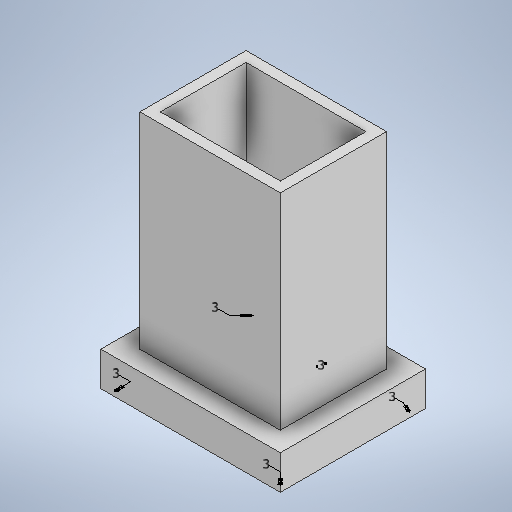
# Autodesk Inventor part: Part3
Saved by Autodesk Inventor 2025.3 (Build 293356000, 356)
## iProperties
Created: 2026-04-30
Part Number: Part3
Material: Generic
Document SubType Name: Modeling
Designer: kamal
Density: 1 g/cm^3
Appearance: Default
Author: kamal
Autodesk Inventor part; units mm, degrees
ref_plane "YZ Plane" through (0, 0, 0) normal (1, 0, 0) x (0, 1, 0)
ref_plane "XZ Plane" through (0, 0, 0) normal (0, 1, 0) x (-1, 0, 0)
ref_plane "XY Plane" through (0, 0, 0) normal (0, 0, 1) x (1, 0, 0)
sketch "Sketch1" plane through (0, 0, 0) normal (0, 1, 0) x (-1, 0, 0)
  line L0 (-17.5, 12.5) -> (17.5, 12.5)
  line L1 (17.5, 12.5) -> (17.5, -12.5)
  line L2 (17.5, -12.5) -> (-17.5, -12.5)
  line L3 (-17.5, -12.5) -> (-17.5, 12.5)
  line L4 (-17.5, 12.5) -> (17.5, -12.5) construction
  line L5 (17.5, 12.5) -> (-17.5, -12.5) construction
  line L6 (26.2, -21.2) -> (-26.2, -21.2)
  line L7 (-26.2, -21.2) -> (-26.2, 21.2)
  line L8 (-26.2, 21.2) -> (26.2, 21.2)
  line L9 (26.2, 21.2) -> (26.2, -21.2)
  line L10 (26.2, -21.2) -> (-26.2, 21.2) construction
  line L11 (-26.2, -21.2) -> (26.2, 21.2) construction
  line L12 (20.5, 15.5) -> (-20.5, 15.5)
  line L13 (-20.5, 15.5) -> (-20.5, -15.5)
  line L14 (-20.5, -15.5) -> (20.5, -15.5)
  line L15 (20.5, -15.5) -> (20.5, 15.5)
  point P0 (0, 0)
  dimension "d0" = 35
  dimension "d1" = 25
  dimension "d2" = 52.4
  dimension "d3" = 42.4
  dimension "d4" = 3
  constraints: 32 end point, 6 parallel, 4 midpoint, 3 perpendicular, 2 horizontal, 3 other
  measures "d0" distance of L1.end L2.end
  measures "d1" distance of L0.end L1.end
  measures "d2" distance of L7.end L8.end
  measures "d3" distance of L8.end L6.start
  measures "d4" distance between parallel lines of L0 L12
extrude "Extrusion1" add sketch "Sketch1" along normal blind 60 contours L15 L14 L13 L12
extrude "Extrusion2" add sketch "Sketch1" against normal blind 10 contours L6 L7 L8 L9
sketch "Sketch2" plane through (0, -10, 0) normal (0, -1, 0) x (1, 0, 0)
  circle A0 centre (23.5, -18.5) radius 1.5
  line L0 (20.5, 15.5) -> (20.5, -15.5) projected
  line L1 (-20.5, 15.5) -> (20.5, 15.5) projected
  line L2 (-20.5, -15.5) -> (-20.5, 15.5) projected
  line L3 (20.5, -15.5) -> (-20.5, -15.5) projected
  line L4 (17.5, 12.5) -> (-17.5, 12.5) projected
  line L5 (17.5, -12.5) -> (17.5, 12.5) projected
  line L6 (-17.5, -12.5) -> (17.5, -12.5) projected
  line L7 (-17.5, 12.5) -> (-17.5, -12.5) projected
  line L8 (-23.5, -18.5) -> (-23.5, 18.5) construction
  line L9 (-23.5, 18.5) -> (23.5, 18.5) construction
  line L10 (23.5, 18.5) -> (23.5, -18.5) construction
  line L11 (23.5, -18.5) -> (-23.5, -18.5) construction
  circle A1 centre (23.5, 18.5) radius 1.5
  circle A2 centre (-23.5, 18.5) radius 1.5
  circle A3 centre (-23.5, -18.5) radius 1.5
  point P0 (0, 0)
  dimension "d9" = 3
  dimension "d10" = 3
  dimension "d11" = 3
  dimension "d12" = 3
  dimension "d13" = 3
  constraints: 8 end point, 4 centre point, 4 coincident, 3 other
  measures "d9" diameter of A0
  measures "d10" distance between parallel lines of L3 L11
  measures "d11" diameter of A1
  measures "d12" diameter of A2
  measures "d13" diameter of A3
body "Solid1"
